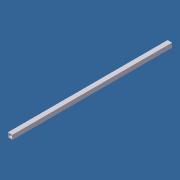
# Autodesk Inventor part: tubing_template_0.125
Saved by Autodesk Inventor 2011 (Build 150239000, 239)
## iProperties
Created: 2010-12-19
Part Number: tubing_template_0.125
Material: Aluminum-6061
Document SubType Name: Modeling
Designer: Antonella Wilby
Mass: 699.441 g
Surface Area: 1631.45 cm^2
Volume: 258.096 cm^3
Density: 2.71 g/cm^3
Author: Antonella Wilby
Autodesk Inventor part; units mm, degrees
ref_plane "YZ Plane" through (0, 0, 0) normal (1, 0, 0) x (0, 1, 0)
ref_plane "XZ Plane" through (0, 0, 0) normal (0, 1, 0) x (-1, 0, 0)
ref_plane "XY Plane" through (0, 0, 0) normal (0, 0, 1) x (1, 0, 0)
sketch "Sketch1" plane through (0, 0, 0) normal (0, 0, 1) x (1, 0, 0)
  line L0 (-17.78, 0) -> (17.78, 0) projected
  line L1 (0, -17.78) -> (0, 17.78) projected
  line L2 (-12.7, 12.7) -> (12.7, 12.7)
  line L3 (12.7, 12.7) -> (12.7, -12.7)
  line L4 (12.7, -12.7) -> (-12.7, -12.7)
  line L5 (-12.7, -12.7) -> (-12.7, 12.7)
  line L6 (9.525, 9.525) -> (-9.525, 9.525)
  line L7 (-9.525, 9.525) -> (-9.525, -9.525)
  line L8 (-9.525, -9.525) -> (9.525, -9.525)
  line L9 (9.525, -9.525) -> (9.525, 9.525)
  point P0 (0, 0)
  point P1 (-12.7, 0)
  point P2 (0, 12.7)
  dimension "d0" = 25.4
  dimension "d1" = 3.175
  constraints: 16 end point, 4 parallel, 3 perpendicular, 2 midpoint, 1 horizontal, 1 horizontal alignment, 1 vertical alignment, 3 other
  measures "d0" distance of L4.end L2.start
  measures "d1" distance between parallel lines of L2 L6
extrude "Extrusion1" add sketch "Sketch1" along normal mid plane 914.4 contours L5 L2 L1 L6 L7 L0 | L0 L7 L8 L1 L4 L5 | L1 L8 L9 L0 L3 L4 | L2 L3 L0 L9 L6 L1
body "Solid1"
